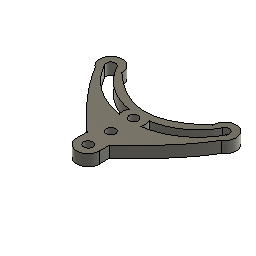
İçi Boş Mıknatıs Tutucu v15 (Autodesk Fusion 360 design; units mm, degrees)
Autodesk Fusion 360 part; units mm, degrees
sketch "Eskiz2" plane through (0, 0, 0) normal (0, 1, 0) x (1, 0, 0)
  circle A0 centre (0, 0) radius 4
  circle A1 centre (0, 0) radius 10
  circle A2 centre (100, 0) radius 10
  circle A3 centre (100, 0) radius 4
  circle A4 centre (50, -50) radius 10
  circle A5 centre (50, -50) radius 4
  circle A6 centre (50, -70) radius 10
  circle A7 centre (50, -70) radius 4
  circle A8 centre (50, -30) radius 4
  circle A9 centre (50, -30) radius 10
  spline S0 degree 5 poles (0, 10) (2, 7.7246) (6, 3.3724) (12, -2.5597) (20, -9.2571) (30, -15.4718) (40, -19.3367) (50, -20.6598) (60, -19.3367) (70, -15.4718) (80, -9.2571) (88, -2.5597) (94, 3.3724) (98, 7.7246) (100, 10) knots 0 0 0 0 0 0 0.1 0.2 0.3 0.4 0.5 0.6 0.7 0.8 0.9 1 1 1 1 1 1
  arc A10 (50, -26) -> (3.5294, 1.8824) centre (50, 26.6667) ccw
  arc A11 (50, -26) -> (50, -34) centre (50, -30) ccw
  arc A12 (50, -34) -> (-3.5294, -1.8824) centre (50, 26.6667) ccw
  arc A13 (-3.5294, -1.8824) -> (3.5294, 1.8824) centre (0, 0) ccw
  arc A14 (50, -30) -> (0, 0) centre (50, 26.6667) ccw construction
  arc A15 (96.4706, 1.8824) -> (50, -26) centre (50, 26.6667) ccw
  arc A16 (96.4706, 1.8824) -> (103.5294, -1.8824) centre (100, 0) ccw
  arc A17 (103.5294, -1.8824) -> (50, -34) centre (50, 26.6667) ccw
  arc A18 (50, -34) -> (50, -26) centre (50, -30) ccw
  arc A19 (100, 0) -> (50, -30) centre (50, 26.6667) ccw construction
  spline S1 degree 5 poles (-10, 0) (-9.333, -1.3072) (-7.9501, -3.9302) (-5.7286, -7.8903) (-2.4678, -13.2224) (2.1378, -19.9797) (7.3113, -26.8359) (13.0844, -33.7964) (19.4493, -40.8599) (26.3611, -48.0186) (33.7681, -55.2635) (40.0526, -61.1218) (44.9543, -65.5484) (48.3044, -68.5137) (50, -70) knots 0 0 0 0 0 0 0.1 0.2 0.3 0.4 0.5 0.6 0.7 0.8 0.9 1 1 1 1 1 1
  spline S2 degree 5 poles (110, 0) (109.333, -1.3072) (107.9501, -3.9302) (105.7286, -7.8903) (102.4678, -13.2224) (97.8622, -19.9797) (92.6887, -26.8359) (86.9156, -33.7964) (80.5507, -40.8599) (73.6389, -48.0186) (66.2319, -55.2635) (59.9474, -61.1218) (55.0457, -65.5484) (51.6956, -68.5137) (50, -70) knots 0 0 0 0 0 0 0.1 0.2 0.3 0.4 0.5 0.6 0.7 0.8 0.9 1 1 1 1 1 1
  spline S3 degree 5 poles (40.5459, -33.2588) (40.5241, -34.7285) (40.4804, -37.6678) (40.4149, -42.0767) (40.3275, -47.9553) (40.2184, -55.3035) (40.131, -61.1821) (40.0655, -65.5911) (40.0218, -68.5304) (40, -70) knots 0 0 0 0 0 0 0.2 0.4 0.6 0.8 1 1 1 1 1 1
  spline S4 degree 5 poles (60, -70) (59.9782, -68.5304) (59.9345, -65.5911) (59.869, -61.1821) (59.7816, -55.3035) (59.6725, -47.9553) (59.5851, -42.0767) (59.5196, -37.6678) (59.4759, -34.7285) (59.4541, -33.2588) knots 0 0 0 0 0 0 0.2 0.4 0.6 0.8 1 1 1 1 1 1
  point P0 (0, -45)
  point P1 (0, -70)
  point P2 (50, -80)
  point P3 (25, -70)
  point P4 (40, -70)
  point P5 (60, -70)
  point P6 (50, 0)
  point P7 (50, -20)
  point P8 (10, -30)
  point P9 (90, -30)
  point P10 (75, -70)
  point P11 (10, -30)
  point P12 (90, -30)
  dimension "d33" = 8
  dimension "d34" = 20
  dimension "d35" = 8
  dimension "d36" = 20
  dimension "d45" = 100
  dimension "d46" = 8
  dimension "d47" = 20
  dimension "d66" = 8
  dimension "d67" = 20
  dimension "d96" = 8
  dimension "d97" = 20
  dimension "d98" = 20
  dimension "d99" = 30
  dimension "d100" = 40
  dimension "d101" = 40
  dimension "d102" = 8
  dimension "d103" = 8
  dimension "d104" = 25
  constraint coincident A0.centre A1.centre
  constraint concentric A0 A1
  constraint concentric A2 A3
  constraint concentric A4 A5
  constraint concentric A6 A7
  constraint coincident A6 P2
  constraint coincident A6 P4
  constraint coincident A6 P5
  constraint concentric A8 A9
  constraint coincident A1 S0.start
  constraint coincident A9 P7
  constraint coincident A2 S0.end
  constraint tangent A10 A11
  constraint tangent A11 A12
  constraint tangent A12 A13
  constraint tangent A10 A13
  constraint coincident A8.centre A9.centre
  constraint tangent A15 A16
  constraint tangent A16 A17
  constraint tangent A17 A18
  constraint tangent A15 A18
  constraint coincident A2.centre A3.centre
  constraint coincident A1 S1.start
  constraint coincident P11 P8
  constraint coincident A6.centre A7.centre
  constraint coincident A2 S2.start
  constraint coincident P12 P9
  constraint coincident A9 S3.start
  constraint coincident A17 S3.start
  constraint coincident P4 S3.end
  constraint coincident P5 S4.start
  constraint coincident A9 S4.end
  constraint coincident A12 S4.end
  measures "d33" diameter of A0
  measures "d34" diameter of A1
  measures "d35" diameter of A3
  measures "d36" diameter of A2
  measures "d45" distance of A0.centre A2.centre
  measures "d46" diameter of A5
  measures "d47" diameter of A4
  measures "d66" diameter of A7
  measures "d67" diameter of A6
  measures "d96" diameter of A8
  measures "d97" diameter of A9
  measures "d98" distance of A4.centre A8.centre
  measures "d99" distance of A8.centre P6
  measures "d100" distance of A8.centre P11
  measures "d101" distance of A8.centre P12
  measures "d102" diameter of A11
  measures "d103" diameter of A16
  measures "d104" distance of A6.centre P10
extrude "Ekstrüde Et2" add sketch "Eskiz2" along normal blind 10 contours A0 A1 S0 A10 A12 A15 A17 | A1 S0 A10 A15 | A1 A12 A17 S1 | A1 S0 A10 A15 | A1 A9 S0 A15 | A1 A4 A17 S1 S3 | A8 A9 A11 A15 A17 | A9 A10 A15 | A1 S1 | A2 A3 S0 A10 A12 A15 A17 | A2 A12 A17 S2 | A9 A12 A17 | A4 A9 S3 | A2 A9 S0 A10 | A2 S0 A10 A15 | A2 S0 A10 A15 | A8 A9 A10 A12 A18 | A2 S2 | A4 A6 S1 S3 | A6 S1 S3 | A4 A9 S4 | A4 S3 S4 | A4 S3 | A2 S0 A10 A15 | A2 A4 A12 S2 S4 | A6 A7 S1 S2 S3 S4 | A6 A7 S1 S2 | A6 S3 | A4 S4 | A6 S2 S4 | A4 A6 S2 S4 | A6 S4 picked at (7.1423, -1.8575) picked at (6.3904, 6.2)
